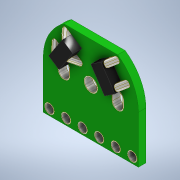
# Autodesk Inventor part: Pololu_Encoder
Saved by Autodesk Inventor 2020 (Build 240168000, 168)
## iProperties
Created: 2020-03-21
Part Number: Pololu_Encoder
Material: Generic
Document SubType Name: Modeling
Designer: ermoz
Density: 1 g/cm^3
Appearance: Default
Author: ermoz
Autodesk Inventor part; units mm, degrees
ref_plane "YZ Plane" through (0, 0, 0) normal (1, 0, 0) x (0, 1, 0)
ref_plane "XZ Plane" through (0, 0, 0) normal (0, 1, 0) x (-1, 0, 0)
ref_plane "XY Plane" through (0, 0, 0) normal (0, 0, 1) x (1, 0, 0)
sketch "Sketch1" plane through (0, 0, 0) normal (0, 0, 1) x (1, 0, 0)
  line L0 (5.75, -5.25) -> (-5.75, -5.25)
  line L1 (-5.75, -5.25) -> (-5.75, 5.25)
  line L2 (-5.75, 5.25) -> (5.75, 5.25)
  line L3 (5.75, 5.25) -> (5.75, -5.25)
  line L4 (5.75, -5.25) -> (-5.75, 5.25) construction
  line L5 (-5.75, -5.25) -> (5.75, 5.25) construction
  line L6 (0, 5.25) -> (3.25, 5.25)
  line L7 (0, 5.25) -> (-3.25, 5.25)
  line L8 (0, 5.25) -> (0, 1.25)
  circle A0 centre (0, 0.5) radius 0.75
  line L9 (0, 0.5) -> (5.75, 0.5)
  circle A1 centre (0, 0.5) radius 5.75
  point P0 (0, 0)
  point P1 (-3.24037, 5.25)
  point P2 (-5.75, 0.5)
  point P3 (3.24037, 5.25)
  dimension "d0" = 11.5
  dimension "d1" = 10.5
  dimension "d3" = 3.25
  constraints: 20 end point, 3 midpoint, 3 perpendicular, 3 point on line, 2 parallel, 1 coincident, 1 horizontal, 1 vertical alignment, 5 other
  measures "d0" distance of L1.end L2.end
  measures "d1" distance of L0.end L1.end
  measures "d3" distance of L6.start L7.end
sketch "Sketch1 outline for Extrusion1" plane through (0, 0, 0) normal (0, 0, 1) x (1, 0, 0)
  line L0 (3.24037, 5.25) -> (-3.24037, 5.25)
  arc A0 (5.75, 0.5) -> (3.24037, 5.25) centre (0, 0.5) ccw
  arc A1 (-3.24037, 5.25) -> (-5.75, 0.5) centre (0, 0.5) ccw
  line L1 (5.75, -5.25) -> (5.75, 0.5)
  line L2 (-5.75, 0.5) -> (-5.75, -5.25)
  line L3 (-5.75, -5.25) -> (5.75, -5.25)
  circle A2 centre (0, 0.5) radius 0.75
extrude "Extrusion1" add sketch "Sketch1 outline for Extrusion1" along normal blind 0.9
sketch "Sketch2" plane through (0, 0, 0.9) normal (0, 0, 1) x (1, 0, 0)
  circle A0 centre (0, 0.5) radius 0.75
  line L0 (5.75, -5.25) -> (5.75, 0.5)
  line L1 (0.75, 0.5) -> (5.75, 0.5)
  line L2 (3.25, 0.125) -> (3.25, 0.875) construction
  line L3 (3.875, 0.125) -> (3.875, 0.875)
  line L4 (2.625, 0.875) -> (2.625, 0.125)
  arc A1 (2.625, 0.125) -> (3.875, 0.125) centre (3.25, 0.125) ccw
  arc A2 (3.875, 0.875) -> (2.625, 0.875) centre (3.25, 0.875) ccw
  line L5 (0, 1.25) -> (0, 2.352119)
  line L6 (-3.25, 0.125) -> (-3.25, 0.875) construction
  line L7 (-3.875, 0.125) -> (-3.875, 0.875)
  line L8 (-2.625, 0.875) -> (-2.625, 0.125)
  arc A3 (-3.875, 0.125) -> (-2.625, 0.125) centre (-3.25, 0.125) ccw
  arc A4 (-2.625, 0.875) -> (-3.875, 0.875) centre (-3.25, 0.875) ccw
  point P0 (0, 0)
  point P1 (3.25, 0.5)
  point P2 (-3.25, 0.5)
  dimension "d8" = 0.375
  dimension "d9" = 1.25
  constraints: 20 end point, 10 point on circle, 7 symmetric about line, 4 centre point, 4 tangent, 2 midpoint, 1 horizontal, 1 parallel, 1 perpendicular, 1 vertical, 2 other
  measures "d8" distance of point (3.25, 0.5) L2.end
  measures "d9" diameter of A2
sketch "Sketch2 outline for Extrusion2" plane through (0, 0, 0.9) normal (0, 0, 1) x (1, 0, 0)
  arc A0 (-2.625, 0.875) -> (-3.875, 0.875) centre (-3.25, 0.875) ccw
  line L0 (-2.625, 0.125) -> (-2.625, 0.875)
  arc A1 (-3.875, 0.125) -> (-2.625, 0.125) centre (-3.25, 0.125) ccw
  line L1 (-3.875, 0.875) -> (-3.875, 0.125)
  arc A2 (3.875, 0.875) -> (2.625, 0.875) centre (3.25, 0.875) ccw
  line L2 (3.875, 0.125) -> (3.875, 0.875)
  arc A3 (2.625, 0.125) -> (3.875, 0.125) centre (3.25, 0.125) ccw
  line L3 (2.625, 0.875) -> (2.625, 0.125)
extrude "Extrusion2" cut sketch "Sketch2 outline for Extrusion2" against normal blind 0.9
sketch "Sketch3" plane through (0, 0, 0.9) normal (0, 0, 1) x (1, 0, 0)
  circle A0 centre (0, 0.5) radius 0.75 projected
  circle A1 centre (0, 0.5) radius 0.85
  arc A2 (-2.625, 0.875) -> (-3.875, 0.875) centre (-3.25, 0.875) ccw projected
  arc A3 (-3.875, 0.125) -> (-2.625, 0.125) centre (-3.25, 0.125) ccw projected
  line L0 (-3.25, 0.875) -> (-3.25, 0.125) construction
  line L1 (-3.975, 0.875) -> (-3.975, 0.125)
  line L2 (-2.525, 0.125) -> (-2.525, 0.875)
  arc A4 (-2.525, 0.875) -> (-3.975, 0.875) centre (-3.25, 0.875) ccw
  arc A5 (-3.975, 0.125) -> (-2.525, 0.125) centre (-3.25, 0.125) ccw
  arc A6 (3.875, 0.875) -> (2.625, 0.875) centre (3.25, 0.875) ccw projected
  arc A7 (2.625, 0.125) -> (3.875, 0.125) centre (3.25, 0.125) ccw projected
  line L3 (3.25, 0.875) -> (3.25, 0.125) construction
  line L4 (2.525, 0.875) -> (2.525, 0.125)
  line L5 (3.975, 0.125) -> (3.975, 0.875)
  arc A8 (3.975, 0.875) -> (2.525, 0.875) centre (3.25, 0.875) ccw
  arc A9 (2.525, 0.125) -> (3.975, 0.125) centre (3.25, 0.125) ccw
  line L6 (-3.25, 0.875) -> (-3.25, 0.125) construction
  line L7 (-3.875, 0.875) -> (-3.875, 0.125)
  line L8 (-2.625, 0.125) -> (-2.625, 0.875)
  arc A10 (-2.625, 0.875) -> (-3.875, 0.875) centre (-3.25, 0.875) ccw
  arc A11 (-3.875, 0.125) -> (-2.625, 0.125) centre (-3.25, 0.125) ccw
  line L9 (3.25, 0.125) -> (3.25, 0.875) construction
  line L10 (3.875, 0.125) -> (3.875, 0.875)
  line L11 (2.625, 0.875) -> (2.625, 0.125)
  arc A12 (2.625, 0.125) -> (3.875, 0.125) centre (3.25, 0.125) ccw
  arc A13 (3.875, 0.875) -> (2.625, 0.875) centre (3.25, 0.875) ccw
  circle A14 centre (0, 0.5) radius 0.75
  line L12 (-5.75, -5.25) -> (5.75, -5.25) projected
  circle A15 centre (1, -4.5) radius 0.5
  circle A16 centre (3, -4.5) radius 0.5
  circle A17 centre (5, -4.5) radius 0.5
  circle A18 centre (-3, -4.5) radius 0.5
  circle A19 centre (-5, -4.5) radius 0.5
  circle A20 centre (-1, -4.5) radius 0.5
  circle A21 centre (-5, -4.5) radius 0.6
  circle A22 centre (-3, -4.5) radius 0.6
  circle A23 centre (-1, -4.5) radius 0.6
  circle A24 centre (1, -4.5) radius 0.6
  circle A25 centre (3, -4.5) radius 0.6
  circle A26 centre (5, -4.5) radius 0.6
  point P0 (0, 0)
  point P1 (-3.25, 0.5)
  point P2 (3.25, 0.5)
  point P3 (-3.25, 0.5)
  point P4 (3.25, 0.5)
  point P5 (2.625, 0.875)
  point P6 (3.875, 0.125)
  point P7 (-3.875, 0.875)
  point P8 (-2.625, 0.125)
  dimension "d12" = 1.7
  dimension "d13" = 1.45
  dimension "d14" = 1.45
  dimension "d26" = 1
  dimension "d27" = 1
  dimension "d28" = 1
  dimension "d29" = 1
  dimension "d30" = 1.2
  dimension "d31" = 1.2
  dimension "d32" = 1.2
  dimension "d33" = 1.2
  dimension "d34" = 1.2
  dimension "d35" = 1.2
  constraints: 32 end point, 22 centre point, 16 point on circle, 16 tangent, 9 coincident, 6 equal length, 4 midpoint, 3 concentric, 2 vertical
  measures "d12" diameter of A1
  measures "d13" diameter of A5
  measures "d14" diameter of A9
  measures "d26" diameter of A15
  measures "d27" diameter of A16
  measures "d28" diameter of A17
  measures "d29" diameter of A20
  measures "d30" diameter of A21
  measures "d31" diameter of A22
  measures "d32" diameter of A23
  measures "d33" diameter of A24
  measures "d34" diameter of A25
  measures "d35" diameter of A26
sketch "Sketch3 outline for Extrusion3" plane through (0, 0, 0.9) normal (0, 0, 1) x (1, 0, 0)
  line L0 (2.525, 0.875) -> (2.525, 0.125)
  arc A0 (3.975, 0.875) -> (2.525, 0.875) centre (3.25, 0.875) ccw
  line L1 (3.975, 0.125) -> (3.975, 0.875)
  arc A1 (2.525, 0.125) -> (3.975, 0.125) centre (3.25, 0.125) ccw
  arc A2 (-3.975, 0.125) -> (-2.525, 0.125) centre (-3.25, 0.125) ccw
  line L2 (-3.975, 0.875) -> (-3.975, 0.125)
  arc A3 (-2.525, 0.875) -> (-3.975, 0.875) centre (-3.25, 0.875) ccw
  line L3 (-2.525, 0.125) -> (-2.525, 0.875)
  circle A4 centre (0, 0.5) radius 0.85
  circle A5 centre (5, -4.5) radius 0.6
  circle A6 centre (3, -4.5) radius 0.6
  circle A7 centre (1, -4.5) radius 0.6
  circle A8 centre (-1, -4.5) radius 0.6
  circle A9 centre (-3, -4.5) radius 0.6
  circle A10 centre (-5, -4.5) radius 0.6
extrude "Extrusion3" cut sketch "Sketch3 outline for Extrusion3" against normal blind 0.9
sketch "Sketch3 outline for Extrusion4" plane through (0, 0, 0.9) normal (0, 0, 1) x (1, 0, 0)
  circle A0 centre (3, -4.5) radius 0.6
  circle A1 centre (3, -4.5) radius 0.5
  circle A2 centre (5, -4.5) radius 0.6
  circle A3 centre (5, -4.5) radius 0.5
  circle A4 centre (1, -4.5) radius 0.6
  circle A5 centre (1, -4.5) radius 0.5
  circle A6 centre (-1, -4.5) radius 0.6
  circle A7 centre (-1, -4.5) radius 0.5
  circle A8 centre (-3, -4.5) radius 0.6
  circle A9 centre (-3, -4.5) radius 0.5
  circle A10 centre (-5, -4.5) radius 0.6
  circle A11 centre (-5, -4.5) radius 0.5
  arc A12 (3.975, 0.875) -> (2.525, 0.875) centre (3.25, 0.875) ccw
  line L0 (3.975, 0.125) -> (3.975, 0.875)
  line L1 (2.525, 0.875) -> (2.525, 0.125)
  arc A13 (2.525, 0.125) -> (3.975, 0.125) centre (3.25, 0.125) ccw
  line L2 (2.625, 0.125) -> (2.625, 0.875)
  arc A14 (3.875, 0.125) -> (2.625, 0.125) centre (3.25, 0.125) cw
  line L3 (3.875, 0.875) -> (3.875, 0.125)
  arc A15 (2.625, 0.875) -> (3.875, 0.875) centre (3.25, 0.875) cw
  circle A16 centre (0, 0.5) radius 0.85
  circle A17 centre (0, 0.5) radius 0.75
  arc A18 (-2.525, 0.875) -> (-3.975, 0.875) centre (-3.25, 0.875) ccw
  line L4 (-2.525, 0.125) -> (-2.525, 0.875)
  line L5 (-3.975, 0.875) -> (-3.975, 0.125)
  arc A19 (-3.975, 0.125) -> (-2.525, 0.125) centre (-3.25, 0.125) ccw
  line L6 (-3.875, 0.125) -> (-3.875, 0.875)
  arc A20 (-2.625, 0.125) -> (-3.875, 0.125) centre (-3.25, 0.125) cw
  line L7 (-2.625, 0.875) -> (-2.625, 0.125)
  arc A21 (-3.875, 0.875) -> (-2.625, 0.875) centre (-3.25, 0.875) cw
extrude "Extrusion4" add sketch "Sketch3 outline for Extrusion4" against normal blind 0.9 separate body
sketch "Sketch4" plane through (0, 0, 0.9) normal (0, 0, 1) x (1, 0, 0)
  circle A0 centre (0, 0.5) radius 0.75
  line L0 (0, 1.25) -> (2.75, 1.25)
  line L1 (0, 1.25) -> (-2.75, 1.25)
  line L2 (0, 1.25) -> (0, 3.75)
  line L3 (2.75, 1.25) -> (1.091688, 3.75)
  line L4 (1.091688, 3.75) -> (2.341688, 4.579156)
  line L5 (2.341688, 4.579156) -> (4, 2.079156)
  line L6 (4, 2.079156) -> (2.75, 1.25)
  line L7 (-2.75, 1.25) -> (-1.091688, 3.75)
  line L8 (-1.091688, 3.75) -> (-2.341688, 4.579156)
  line L9 (-2.341688, 4.579156) -> (-4, 2.079156)
  line L10 (-4, 2.079156) -> (-2.75, 1.25)
  point P0 (0, 0)
  dimension "d40" = 2.75
  dimension "d41" = 2.75
  dimension "d42" = 2.5
  dimension "d44" = 3
  dimension "d45" = 1.5
  dimension "d46" = 3
  constraints: 22 end point, 3 horizontal, 3 symmetric about line, 2 perpendicular, 1 vertical, 1 vertical alignment, 1 other
  measures "d40" distance of L0.start L0.end
  measures "d41" distance of L0.start L1.end
  measures "d42" distance of L0.start L2.end
  measures "d44" distance of L0.end L3.end
  measures "d45" distance of L3.end L4.end
  measures "d46" distance of L4.end L5.end
sketch "Sketch4 outline for Extrusion5" plane through (0, 0, 0.9) normal (0, 0, 1) x (1, 0, 0)
  line L0 (2.75, 1.25) -> (4, 2.079156)
  line L1 (1.091688, 3.75) -> (2.75, 1.25)
  line L2 (2.341688, 4.579156) -> (1.091688, 3.75)
  line L3 (4, 2.079156) -> (2.341688, 4.579156)
  line L4 (-2.75, 1.25) -> (-1.091688, 3.75)
  line L5 (-4, 2.079156) -> (-2.75, 1.25)
  line L6 (-2.341688, 4.579156) -> (-4, 2.079156)
  line L7 (-1.091688, 3.75) -> (-2.341688, 4.579156)
extrude "Extrusion5" add sketch "Sketch4 outline for Extrusion5" along normal blind 1.1 separate body
sketch "Sketch5" plane through (0, 0, 0.9) normal (0, 0, 1) x (1, 0, 0)
  line L0 (-4, 2.079156) -> (-4.833333, 2.631927)
  line L1 (-4.833333, 2.631927) -> (-4.418755, 3.256927)
  line L2 (-4.418755, 3.256927) -> (-3.585422, 2.704156)
  line L3 (-3.585422, 2.704156) -> (-4, 2.079156)
  line L4 (-4, 2.079156) -> (-2.75, 1.25)
  line L5 (-2.341688, 4.579156) -> (-3.175021, 5.131927)
  line L6 (-3.175021, 5.131927) -> (-3.589599, 4.506927)
  line L7 (-3.589599, 4.506927) -> (-2.756266, 3.954156)
  line L8 (-2.756266, 3.954156) -> (-2.341688, 4.579156)
  line L9 (-1.091688, 3.75) -> (-2.341688, 4.579156)
  line L10 (-2.75, 1.25) -> (-1.091688, 3.75)
  line L11 (-1.920844, 2.5) -> (-1.713555, 2.8125)
  line L12 (-1.713555, 2.8125) -> (-0.880221, 2.259729)
  line L13 (-0.880221, 2.259729) -> (-1.2948, 1.634729)
  line L14 (-1.2948, 1.634729) -> (-2.128133, 2.1875)
  line L15 (-2.128133, 2.1875) -> (-1.713555, 2.8125)
  circle A0 centre (0, 0.5) radius 0.85
  line L16 (0, 1.35) -> (0, 2.125856)
  line L17 (4, 2.079156) -> (4.833333, 2.631927)
  line L18 (4.833333, 2.631927) -> (4.418755, 3.256927)
  line L19 (4.418755, 3.256927) -> (3.585422, 2.704156)
  line L20 (3.585422, 2.704156) -> (4, 2.079156)
  line L21 (4, 2.079156) -> (2.75, 1.25)
  line L22 (2.341688, 4.579156) -> (3.175021, 5.131927)
  line L23 (3.175021, 5.131927) -> (3.589599, 4.506927)
  line L24 (3.589599, 4.506927) -> (2.756266, 3.954156)
  line L25 (2.756266, 3.954156) -> (2.341688, 4.579156)
  line L26 (1.091688, 3.75) -> (2.341688, 4.579156)
  line L27 (2.75, 1.25) -> (1.091688, 3.75)
  line L28 (1.920844, 2.5) -> (1.713555, 2.8125)
  line L29 (1.713555, 2.8125) -> (0.880221, 2.259729)
  line L30 (0.880221, 2.259729) -> (1.2948, 1.634729)
  line L31 (1.2948, 1.634729) -> (2.128133, 2.1875)
  line L32 (2.128133, 2.1875) -> (1.713555, 2.8125)
  point P0 (0, 0)
  dimension "d50" = 1
  dimension "d51" = 0.75
  dimension "d52" = 1
  dimension "d53" = 0.75
  dimension "d54" = 0.375
  dimension "d55" = 1
  dimension "d56" = 0.75
  constraints: 60 end point, 15 symmetric about line, 7 parallel, 3 perpendicular, 2 collinear, 2 point on line, 1 midpoint, 1 vertical, 1 vertical alignment, 1 other
  measures "d50" distance of L0.start L0.end
  measures "d51" distance of L0.end L1.end
  measures "d52" distance of L5.start L5.end
  measures "d53" distance of L6.end L5.end
  measures "d54" distance of L11.start L11.end
  measures "d55" distance of L11.end L12.end
  measures "d56" distance of L12.end L13.end
sketch "Sketch5 outline for Extrusion6" plane through (0, 0, 0.9) normal (0, 0, 1) x (1, 0, 0)
  line L0 (4, 2.079156) -> (4.833333, 2.631927)
  line L1 (3.585422, 2.704156) -> (4, 2.079156)
  line L2 (4.418755, 3.256927) -> (3.585422, 2.704156)
  line L3 (4.833333, 2.631927) -> (4.418755, 3.256927)
  line L4 (2.341688, 4.579156) -> (2.756266, 3.954156)
  line L5 (3.175021, 5.131927) -> (2.341688, 4.579156)
  line L6 (3.589599, 4.506927) -> (3.175021, 5.131927)
  line L7 (2.756266, 3.954156) -> (3.589599, 4.506927)
  line L8 (0.880221, 2.259729) -> (1.2948, 1.634729)
  line L9 (1.713555, 2.8125) -> (0.880221, 2.259729)
  line L10 (2.128133, 2.1875) -> (1.713555, 2.8125)
  line L11 (1.2948, 1.634729) -> (2.128133, 2.1875)
  line L12 (-1.2948, 1.634729) -> (-0.880221, 2.259729)
  line L13 (-2.128133, 2.1875) -> (-1.2948, 1.634729)
  line L14 (-1.713555, 2.8125) -> (-2.128133, 2.1875)
  line L15 (-0.880221, 2.259729) -> (-1.713555, 2.8125)
  line L16 (-4, 2.079156) -> (-3.585422, 2.704156)
  line L17 (-4.833333, 2.631927) -> (-4, 2.079156)
  line L18 (-4.418755, 3.256927) -> (-4.833333, 2.631927)
  line L19 (-3.585422, 2.704156) -> (-4.418755, 3.256927)
  line L20 (-2.341688, 4.579156) -> (-3.175021, 5.131927)
  line L21 (-2.756266, 3.954156) -> (-2.341688, 4.579156)
  line L22 (-3.589599, 4.506927) -> (-2.756266, 3.954156)
  line L23 (-3.175021, 5.131927) -> (-3.589599, 4.506927)
extrude "Extrusion6" add sketch "Sketch5 outline for Extrusion6" along normal blind 0.9 bodies 2
sketch "Sketch6" plane through (-4, 2.079156, 0.9) normal (-0.5527708, -0.8333333, 0) x (0.8333333, -0.5527708, 0)
  line L0 (-1, 0) -> (-1, 0.9) projected
  line L1 (0, 0.9) -> (-1, 0.9) projected
  line L2 (-1, 0) -> (0, 0.9)
  line L3 (0, 0.9) -> (-1, 0.9)
  line L4 (-1, 0.9) -> (-1, 0)
  line L5 (1.5, 0) -> (1.5, 1.1) projected
  line L6 (2.5, 0) -> (2.5, 0.9) projected
  line L7 (1.5, 0.9) -> (2.5, 0)
  line L8 (1.5, 0.9) -> (2.5, 0.9) projected
  line L9 (2.5, 0) -> (2.5, 0.9)
  line L10 (2.5, 0.9) -> (1.5, 0.9)
  point P0 (4.48263, -0.9)
  constraints: 12 end point, 3 perpendicular, 2 point on line, 1 collinear
sketch "Sketch6 outline for Extrusion7" plane through (-4, 2.079156, 0.9) normal (-0.5527708, -0.8333333, 0) x (0.8333333, -0.5527708, 0)
  line L0 (-1, 0) -> (0, 0.9)
  line L1 (-1, 0.9) -> (-1, 0)
  line L2 (0, 0.9) -> (-1, 0.9)
  line L3 (2.5, 0.9) -> (1.5, 0.9)
  line L4 (2.5, 0) -> (2.5, 0.9)
  line L5 (1.5, 0.9) -> (2.5, 0)
extrude "Extrusion7" cut sketch "Sketch6 outline for Extrusion7" against normal blind 5 bodies 2
sketch "Sketch7" plane through (4.833333, 2.631927, 0.9) normal (0.5527708, -0.8333333, 0) x (0.8333333, 0.5527708, 0)
  line L0 (-1, 0.9) -> (0, 0.9) projected
  line L1 (0, 0) -> (0, 0.9) projected
  line L2 (-1, 0.9) -> (0, 0)
  line L3 (0, 0) -> (0, 0.9)
  line L4 (0, 0.9) -> (-1, 0.9)
  line L5 (-2.5, 0.9) -> (-3.5, 0.9) projected
  line L6 (-3.5, 0) -> (-3.5, 0.9) projected
  line L7 (-2.5, 0.9) -> (-3.5, 0)
  line L8 (-3.5, 0) -> (-3.5, 0.9)
  line L9 (-3.5, 0.9) -> (-2.5, 0.9)
  point P0 (-5.48263, -0.9)
  constraints: 12 end point, 3 perpendicular, 1 point on line, 1 vertical
sketch "Sketch7 outline for Extrusion8" plane through (4.833333, 2.631927, 0.9) normal (0.5527708, -0.8333333, 0) x (0.8333333, 0.5527708, 0)
  line L0 (-3.5, 0) -> (-2.5, 0.9)
  line L1 (-3.5, 0.9) -> (-3.5, 0)
  line L2 (-2.5, 0.9) -> (-3.5, 0.9)
  line L3 (-1, 0.9) -> (0, 0)
  line L4 (0, 0.9) -> (-1, 0.9)
  line L5 (0, 0) -> (0, 0.9)
extrude "Extrusion8" cut sketch "Sketch7 outline for Extrusion8" against normal blind 5 bodies 2
fillet "Fillet1" radius 0.25 12 edges at (-1.7115, 1.9111, 1.35) (-1.2969, 2.5361, 1.35) (1.7115, 1.9111, 1.35) (1.2969, 2.5361, 1.35) (4.4167, 2.3555, 1.35) (4.0021, 2.9805, 1.35) (3.1729, 4.2305, 1.35) (2.7584, 4.8555, 1.35) (-4.4167, 2.3555, 1.35) (-4.0021, 2.9805, 1.35) (-3.1729, 4.2305, 1.35) (-2.7584, 4.8555, 1.35)
body "Solid1"
body "Solid2"
body "Solid3"
